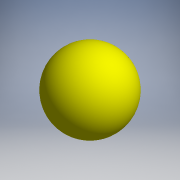
# Autodesk Inventor part: 30-62-38.1-18-ybrg1-619.525-46-b
Saved by Autodesk Inventor 2017.3 (Build 213256000, 256)
## iProperties
Part Number: 30-62-38.1-18-ybrg1-619.525-46-b
Material: Generic
Catalog Web Link: www.cadenas.de
Description: ayp_001_hc_hh_hy-ayl_001_hp_ball-Y-bearings
Vendor: SKF
Document SubType Name: Modeling
Designer: partserver
Manufacturer: SKF
Mass: 0.452474 g
Surface Area: 2.85023 cm^2
Volume: 0.452474 cm^3
Density: 1 g/cm^3
Appearance: PSOLRGB-255-255-0
Category: PARTsolutions
Company: SKF
Title: 30-62-38.1-18-ybrg1-619.525-46-b
Author: Cadenas PARTsolutions
Comments: Y-bearings
PSOL_IDENT_0: {$CADENAS_DATA\23d-libs\skf\bearings_units_and_housings\bearing_units\ball_bearing_units\y-units\y-b
PSOL_IDENT_1: earing_plummer_block_units_parts\ayp_001_hc_hh_hy-ayl_001_hp_ball.prj},232 {VTYP=3D},{NB=30-62-38.1-
PSOL_IDENT_2: 18-ybrg1-619.525-46-b},{LINA=30-62-38.1-18-ybrg1-619.525-46-b},{NN=ayp_001_hc_hh_hy-ayl_001_hp_ball}
PSOL_IDENT_3: ,{DATE=17.09.2021 07:33:22},{GEOMDATE=16.12.2020 09:40:00},{VERSION=},{LINEID=1580},{WBVAR=},{WBNUME
PSOL_IDENT_4: RIC=}  {NB=30-62-38.1-18-ybrg1-619.525-46-b},{LINA=30-62-38.1-18-ybrg1-619.525-46-b},{KT=DUMMY},{DD=
PSOL_IDENT_5: 30.0000},{D=62},{B=38.100},{C=18.000},{PITCH=46.000},{DW=9.525},{FO=IEC_BBY_006},{DESIGN=ybrg1},{X=0
PSOL_IDENT_6: },{PN=61}
NB: 30-62-38.1-18-ybrg1-619.525-46-b
NN: ayp_001_hc_hh_hy-ayl_001_hp_ball
NT: Y-bearings
NBSYN: $DD.-$D.-$B.-$C.-$DESIGN.-$PN.$DW.-$PITCH.-b
LINA: 30-62-38.1-18-ybrg1-619.525-46-b
CATALOG: SKF
DD: 30
D: 62
B: 38.1
C: 18
PITCH: 46
DW: 9.525
FO: IEC_BBY_006
DESIGN: ybrg1
PN: 61
SUPPLIER: SKF
ARTICLENO: 30-62-38.1-18-ybrg1-619.525-46-b
BOMINFO: 30-62-38.1-18-ybrg1-619.525-46-b
CREATOR: CADENAS GmbH
Autodesk Inventor part; units mm, degrees
sketch "Sketch_1" plane through (0, 0, 0) normal (0, 0, 1) x (1, 0, 0)
  line L0 (4.7625, 23) -> (-4.7625, 23)
  arc A0 (4.7625, 23) -> (-4.7625, 23) centre (0, 23) ccw
  line L1 (4.7625, 23) -> (-4.7625, 23)
  constraints: 4 end point, 2 point on circle, 1 centre point
revolve "Revolution1" add sketch "Sketch_1" angle 360 about axis through (4.7625, 23, 0) along (1, 0, 0)
ref_plane "ball_XY" through (0, 23, 0) normal (1, 0, 0) x (0, 0, -1)
ref_plane "ball_YZ" through (0, 23, 0) normal (0, 0, -1) x (0, 1, 0)
ref_plane "ball_ZX" through (0, 23, 0) normal (0, 1, 0) x (1, 0, 0)
body "Solid1"
